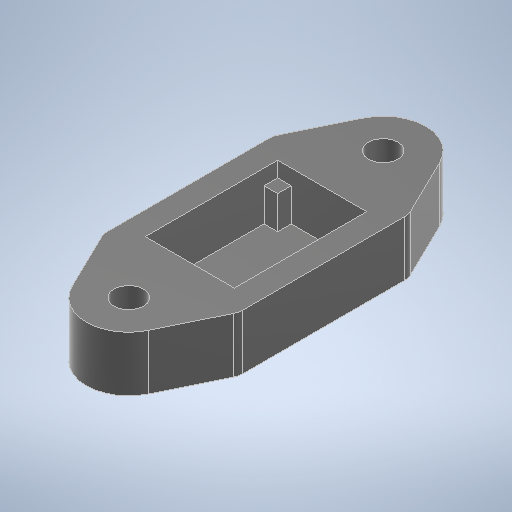
# Autodesk Inventor part: 3D_bno055_top
Saved by Autodesk Inventor 2025.1 (Build 291241020, 241B)
## iProperties
Created: 2024-08-31
Part Number: 3D_bno055_top
Material: 一般
Document SubType Name: Modeling
Designer: 8326d
Density: 1 g/cm^3
Appearance: 滑らか - 黒
Author: 8326d
## iProperties of the stored document 3D_bno055_top_3D プリント.ipt
Created: 2024-09-02
Part Number: 3D_bno055_top_3D プリント
Material: 一般
Document SubType Name: Modeling
Designer: 8326d
Density: 1 g/cm^3
Appearance: 既定
Author: 8326d
Autodesk Inventor part; units mm, degrees
ref_plane "YZ Plane" through (0, 0, 0) normal (1, 0, 0) x (0, 1, 0)
ref_plane "XZ Plane" through (0, 0, 0) normal (0, 1, 0) x (-1, 0, 0)
ref_plane "XY Plane" through (0, 0, 0) normal (0, 0, 1) x (1, 0, 0)
sketch "スケッチ1" plane through (0, 0, 0) normal (0, 1, 0) x (-1, 0, 0)
  line L0 (-8, 10) -> (8, 10)
  line L1 (8, 10) -> (8, -10)
  line L2 (8, -10) -> (-8, -10)
  line L3 (-8, -10) -> (-8, 10)
  line L4 (-8, 10) -> (8, -10) construction
  line L5 (8, 10) -> (-8, -10) construction
  circle A0 centre (0, 15) radius 5
  circle A1 centre (0, -15) radius 5
  line L6 (4.4944, 17.191) -> (8, 10)
  line L7 (-8, 10) -> (-4.4944, 17.191)
  line L8 (4.4944, -17.191) -> (8, -10)
  line L9 (-8, -10) -> (-4.4944, -17.191)
  point P0 (0, 0)
  dimension "d0" = 16
  dimension "d1" = 20
  dimension "d2" = 10
  dimension "d3" = 10
  constraints: 20 end point, 6 tangent, 4 point on circle, 2 centre point, 2 midpoint, 2 parallel, 2 vertical alignment, 1 horizontal, 1 perpendicular
  measures "d0" distance of L1.end L2.end
  measures "d1" distance of L0.end L1.end
  measures "d2" diameter of A0
  measures "d3" diameter of A1
extrude "押し出し1" add sketch "スケッチ1" along normal blind 6.5
sketch "スケッチ2" plane through (0, 6.5, 0) normal (0, 1, 0) x (1, 0, 0)
  line L0 (5.25, -7.8) -> (-5.25, -7.8)
  line L1 (-5.25, -7.8) -> (-5.25, 7.8)
  line L2 (-5.25, 7.8) -> (5.25, 7.8)
  line L3 (5.25, 7.8) -> (5.25, -7.8)
  line L4 (5.25, -7.8) -> (-5.25, 7.8) construction
  line L5 (-5.25, -7.8) -> (5.25, 7.8) construction
  point P0 (0, 0)
  dimension "d6" = 10.5
  dimension "d7" = 15.6
  constraints: 12 end point, 2 midpoint, 2 parallel, 1 horizontal, 1 perpendicular
  measures "d6" distance of L1.end L2.end
  measures "d7" distance of L0.end L1.end
extrude "押し出し2" cut sketch "スケッチ2" against normal blind 1.8
sketch "スケッチ3" plane through (0, 4.7, 0) normal (0, 1, 0) x (1, 0, 0)
  line L0 (-5.25, 7.8) -> (5.25, 7.8) projected
  line L1 (-5.25, -7.8) -> (-5.25, 7.8) projected
  line L2 (5.25, -7.8) -> (-5.25, -7.8) projected
  line L3 (5.25, 7.8) -> (5.25, -7.8) projected
  line L4 (-5.25, -7.8) -> (-3.65, -7.8)
  line L5 (-3.65, -7.8) -> (-3.65, -6.2)
  line L6 (-3.65, -6.2) -> (-5.25, -6.2)
  line L7 (-5.25, -6.2) -> (-5.25, -7.8)
  line L8 (5.25, -7.8) -> (3.65, -7.8)
  line L9 (3.65, -7.8) -> (3.65, -6.2)
  line L10 (3.65, -6.2) -> (5.25, -6.2)
  line L11 (5.25, -6.2) -> (5.25, -7.8)
  line L12 (-5.25, 7.8) -> (-3.65, 7.8)
  line L13 (-3.65, 7.8) -> (-3.65, 6.2)
  line L14 (-3.65, 6.2) -> (-5.25, 6.2)
  line L15 (-5.25, 6.2) -> (-5.25, 7.8)
  line L16 (-5.25, 7.8) -> (5.25, 7.8) projected
  line L17 (5.25, 7.8) -> (3.65, 7.8)
  line L18 (3.65, 7.8) -> (3.65, 6.2)
  line L19 (3.65, 6.2) -> (5.25, 6.2)
  line L20 (5.25, 6.2) -> (5.25, 7.8)
  point P0 (0, 0)
  point P1 (-5.25, 6.2)
  point P2 (3.65, -7.8)
  dimension "d10" = 1.6
  dimension "d11" = 1.6
  dimension "d12" = 1.6
  dimension "d13" = 1.6
  dimension "d14" = 1.6
  dimension "d15" = 1.6
  dimension "d16" = 1.6
  dimension "d17" = 1.6
  constraints: 32 end point, 8 parallel, 4 horizontal, 4 perpendicular
  measures "d10" distance of L6.end L5.end
  measures "d11" distance of L5.end L4.end
  measures "d12" distance of L9.end L10.end
  measures "d13" distance of L8.end L9.end
  measures "d14" distance of L13.end L14.end
  measures "d15" distance of L12.end L13.end
  measures "d16" distance of L19.end L18.end
  measures "d17" distance of L18.end L17.end
extrude "押し出し3" cut sketch "スケッチ3" against normal blind 3.9 contours L0 L18 L19 L3 L10 L9 L2 L5 L6 L1 L14 L13
sketch "スケッチ4" plane through (0, 6.5, 0) normal (0, 1, 0) x (1, 0, 0)
  arc A0 (-4.4944, -17.191) -> (4.4944, -17.191) centre (0, -15) ccw projected
  arc A1 (4.4944, 17.191) -> (-4.4944, 17.191) centre (0, 15) ccw projected
  point P0 (0, 0)
hole "穴1" at (0, 6.5, 15) at (0, 6.5, -15) direction (0, -1, 0) diameter 3.5 end through all
fillet "フィレット1" radius 2 4 edges at (8, 3.25, 10) (8, 3.25, -10) (-8, 3.25, -10) (-8, 3.25, 10)
sketch "スケッチ5" plane through (0, 0, 0) normal (0, -1, 0) x (1, 0, 0)
  line L0 (3.9393, 10.9499) -> (3.9393, -11.5207) construction
  line L1 (3.9393, -11.5207) -> (-3.7897, -11.5207) construction
  line L2 (-3.7897, -11.5207) -> (-3.7897, 10.9499) construction
  line L3 (-3.7897, 10.9499) -> (3.9393, 10.9499) construction
  line L4 (-3.0607, 6.887) -> (-3.0607, 10.9842)
  line L5 (-3.0607, 10.9842) -> (-1.8207, 10.6984)
  line L6 (-1.8207, 10.6984) -> (-1.8207, 9.5556)
  line L7 (-1.8207, 9.5556) -> (2.6993, 8.5156)
  line L8 (2.6993, 8.5156) -> (2.6993, 9.6584)
  line L9 (2.6993, 9.6584) -> (3.9393, 9.367)
  line L10 (3.9393, 9.367) -> (3.9393, 5.2699)
  line L11 (3.9393, 5.2699) -> (2.6993, 5.5556)
  line L12 (2.6993, 5.5556) -> (2.6993, 6.6984)
  line L13 (2.6993, 6.6984) -> (-1.8207, 7.7442)
  line L14 (-1.8207, 7.7442) -> (-1.8207, 6.6013)
  line L15 (-1.8207, 6.6013) -> (-3.0607, 6.887)
  line L16 (-3.0607, -1.9358) -> (-3.0607, -0.1301)
  line L17 (-3.0607, -0.1301) -> (1.5164, -1.1873)
  line L18 (1.5164, -1.1873) -> (-1.415, 0.7327)
  line L19 (-1.415, 0.7327) -> (-1.415, 1.9784)
  line L20 (-1.415, 1.9784) -> (1.7107, 2.6013)
  line L21 (1.7107, 2.6013) -> (-3.0607, 3.6984)
  line L22 (-3.0607, 3.6984) -> (-3.0607, 5.4127)
  line L23 (-3.0607, 5.4127) -> (3.9393, 3.7956)
  line L24 (3.9393, 3.7956) -> (3.9393, 1.7213)
  line L25 (3.9393, 1.7213) -> (0.425, 0.9556)
  line L26 (0.425, 0.9556) -> (3.9393, -1.4216)
  line L27 (3.9393, -1.4216) -> (3.9393, -3.553)
  line L28 (3.9393, -3.553) -> (-3.0607, -1.9358)
  line L29 (3.9393, -11.473) -> (-0.4322, -10.4558)
  spline S0 degree 2 poles (-0.4322, -10.4558) (-1.8836, -10.113) (-3.1979, -8.4787) (-3.1979, -6.9244) knots 0 0 0 1 2 2 2
  spline S1 degree 2 poles (-3.1979, -6.9244) (-3.1979, -5.5416) (-2.2036, -4.1244) (-1.1979, -4.1244) knots 0 0 0 1 2 2 2
  spline S2 degree 2 poles (-1.1979, -4.1244) (-0.9922, -4.1244) (-0.5693, -4.193) (-0.3979, -4.2273) knots 0 0 0 1 2 2 2
  line L30 (-0.3979, -4.2273) -> (3.9393, -5.2387)
  line L31 (3.9393, -5.2387) -> (3.9393, -7.0616)
  line L32 (3.9393, -7.0616) -> (-0.4036, -6.0501)
  spline S3 degree 2 poles (-0.4036, -6.0501) (-0.535, -6.0158) (-0.8493, -5.9758) (-0.9522, -5.9758) knots 0 0 0 1 2 2 2
  spline S4 degree 2 poles (-0.9522, -5.9758) (-1.3922, -5.9758) (-1.8493, -6.5073) (-1.8493, -7.1244) knots 0 0 0 1 2 2 2
  spline S5 degree 2 poles (-1.8493, -7.1244) (-1.8493, -7.7187) (-1.1922, -8.4558) (-0.495, -8.6158) knots 0 0 0 1 2 2 2
  line L33 (-0.495, -8.6158) -> (3.9393, -9.6501)
  line L34 (3.9393, -9.6501) -> (3.9393, -11.473)
  point P0 (0, 0)
  constraints: 2 other
extrude "押し出し4" cut sketch "スケッチ5" against normal blind 0.4
equation "\"d3\" = d2"
